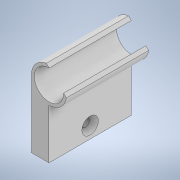
# Autodesk Inventor part: shadeHolderKetchenWindowV2
Saved by Autodesk Inventor 2022 (Build 260153070, 153G)
## iProperties
Created: 2021-02-12
Part Number: shadeHolderKetchenWindowV2
Material: Generic
Document SubType Name: Modeling
Designer: robst
Density: 1 g/cm^3
Appearance: Default
Author: robst
Autodesk Inventor part; units mm, degrees
ref_plane "YZ Plane" through (0, 0, 0) normal (1, 0, 0) x (0, 1, 0)
ref_plane "XZ Plane" through (0, 0, 0) normal (0, 1, 0) x (-1, 0, 0)
ref_plane "XY Plane" through (0, 0, 0) normal (0, 0, 1) x (1, 0, 0)
sketch "Sketch4" plane through (0, 0, 0) normal (0, 0, 1) x (1, 0, 0)
  arc A0 (0.0635, 6.3497) -> (6.3497, 0.0635) centre (0, 0) ccw
  arc A1 (-1.1235, 7.5367) -> (7.5367, -1.1235) centre (0, 0) ccw
  line L0 (0, 0) -> (0, 7.9375) construction
  line L1 (0.0635, 6.3497) -> (6.3497, 0.0635) construction
  line L2 (0.0635, 6.3497) -> (-1.1235, 7.5367)
  line L3 (6.3497, 0.0635) -> (7.5367, -1.1235)
  circle A2 centre (0, 0) radius 6.35
  dimension "d10" = 12.7
  dimension "d11" = 1.27
  dimension "d12" = 45
  dimension "d13" = 8.89
  constraints: 8 end point, 4 point on circle, 3 centre point, 3 coincident, 1 collinear, 1 concentric, 1 point on line, 1 vertical
  measures "d10" diameter of A0
  measures "d11" radial gap between concentric circles of A1 A0
  measures "d12" angle of L1 L0
  measures "d13" distance of L1.start L1.end
extrude "Extrusion3" add sketch "Sketch4" along normal mid plane 35.56 contours A0 L3 A1 L2
sketch "Sketch5" plane through (0, 0, 0) normal (0, 0, 1) x (1, 0, 0)
  arc A0 (-1.1235, 7.5367) -> (7.5367, -1.1235) centre (0, 0) ccw projected
  line L0 (-7.62, 0) -> (-7.62, -29.21)
  line L1 (-7.62, -29.21) -> (0, -29.21)
  line L2 (0, -29.21) -> (0, -7.62)
  circle A1 centre (0, 0) radius 7.9375
  dimension "d16" = 21.59
  constraints: 6 end point, 2 perpendicular, 2 point on circle, 1 centre point, 1 coincident, 1 tangent, 1 vertical
  measures "d16" distance from line of L2.end L1
extrude "Extrusion4" add sketch "Sketch5" along normal mid plane 35.56 contours A0 L2 A1 L0 | A1 L2 L1 L0 picked at (-7.3048, -2.4081)
sketch "Sketch6" plane through (0, -29.21, 17.78) normal (1, 0, 0) x (0, 0, -1)
  line L0 (0, 21.59) -> (35.56, 21.59) projected
  line L1 (35.56, 21.59) -> (35.56, 0) projected
  line L2 (0, 0) -> (35.56, 0) projected
  line L3 (0, 0) -> (0, 21.59) projected
  line L4 (17.78, 0) -> (17.78, 21.59) construction
  point P0 (17.78, 29.21)
  point P1 (17.78, 5.08)
  dimension "d30" = 5.08
  dimension "d31" = 0
  constraints: 2 end point, 2 midpoint
  measures "d30" distance from line of point (17.78, 5.08) L2
  measures "d31" distance from line of point (17.78, 5.08) L4
hole "Hole1" at (0, -24.13, 0) direction (-1, 0, 0) diameter 3.5052 end through all countersink diameter 7.112 countersink angle 82
sketch "Sketch10" plane through (-7.62, -29.21, 17.78) normal (0, -1, 0) x (1, 0, 0)
  line L0 (0, -35.56) -> (0, 0) projected
  line L1 (7.62, -35.56) -> (0, -35.56) projected
  line L2 (7.62, 0) -> (7.62, -35.56) projected
  line L3 (0, 0) -> (7.62, 0) projected
  line L4 (3.81, -35.56) -> (3.81, 0) construction
  line L5 (6.35, -29.5599) -> (1.27, -29.5599)
  line L6 (1.27, -29.5599) -> (1.27, -26.3818)
  line L7 (1.27, -26.3818) -> (1.871, -26.3818)
  line L8 (1.871, -26.3818) -> (1.871, -28.8848)
  line L9 (1.871, -28.8848) -> (3.2625, -28.8848)
  line L10 (3.2625, -28.8848) -> (3.2625, -26.5506)
  line L11 (3.2625, -26.5506) -> (3.8635, -26.5506)
  line L12 (3.8635, -26.5506) -> (3.8635, -28.8848)
  line L13 (3.8635, -28.8848) -> (5.749, -28.8848)
  line L14 (5.749, -28.8848) -> (5.749, -26.3818)
  line L15 (5.749, -26.3818) -> (6.35, -26.3818)
  line L16 (6.35, -26.3818) -> (6.35, -29.5599)
  line L17 (1.27, -19.9474) -> (6.35, -21.2236)
  line L18 (6.35, -21.2236) -> (6.35, -21.9811)
  line L19 (6.35, -21.9811) -> (2.1345, -23.0144)
  line L20 (2.1345, -23.0144) -> (6.35, -24.0188)
  line L21 (6.35, -24.0188) -> (6.35, -24.7681)
  line L22 (6.35, -24.7681) -> (1.27, -26.0648)
  line L23 (1.27, -26.0648) -> (1.27, -25.3691)
  line L24 (1.27, -25.3691) -> (5.4814, -24.3482)
  line L25 (5.4814, -24.3482) -> (1.27, -23.3355)
  line L26 (1.27, -23.3355) -> (1.27, -22.648)
  line L27 (1.27, -22.648) -> (5.5308, -21.6271)
  line L28 (5.5308, -21.6271) -> (1.27, -20.6102)
  line L29 (1.27, -20.6102) -> (1.27, -19.9474)
  line L30 (4.4357, -17.6256) -> (4.4357, -19.5481)
  line L31 (4.4357, -19.5481) -> (3.8182, -19.5481)
  line L32 (3.8182, -19.5481) -> (3.8182, -17.6256)
  line L33 (3.8182, -17.6256) -> (4.4357, -17.6256)
  spline S0 degree 2 poles (2.8014, -13.5954) (3.1307, -13.5954) (3.7235, -13.83) (3.9294, -14.04) knots 0 0 0 1 2 2 2
  spline S1 degree 2 poles (3.9294, -14.04) (4.1887, -14.3035) (4.4563, -15.0156) (4.4563, -15.559) knots 0 0 0 1 2 2 2
  line L34 (4.4563, -15.559) -> (4.4563, -16.1313)
  line L35 (4.4563, -16.1313) -> (6.35, -16.1313)
  line L36 (6.35, -16.1313) -> (6.35, -16.8064)
  line L37 (6.35, -16.8064) -> (1.27, -16.8064)
  line L38 (1.27, -16.8064) -> (1.27, -15.5302)
  spline S2 degree 2 poles (1.27, -15.5302) (1.27, -15.0774) (1.4182, -14.4434) (1.587, -14.2005) knots 0 0 0 1 2 2 2
  spline S3 degree 2 poles (1.587, -14.2005) (1.7805, -13.9165) (2.3774, -13.5954) (2.8014, -13.5954) knots 0 0 0 1 2 2 2
  spline S4 degree 2 poles (2.822, -14.2993) (2.5585, -14.2993) (2.1716, -14.4805) (2.0481, -14.6657) knots 0 0 0 1 2 2 2
  spline S5 degree 2 poles (2.0481, -14.6657) (1.941, -14.8263) (1.8546, -15.2544) (1.8546, -15.5714) knots 0 0 0 1 2 2 2
  line L39 (1.8546, -15.5714) -> (1.8546, -16.1313)
  line L40 (1.8546, -16.1313) -> (3.88, -16.1313)
  line L41 (3.88, -16.1313) -> (3.88, -15.6702)
  spline S6 degree 2 poles (3.88, -15.6702) (3.88, -15.2585) (3.7482, -14.7522) (3.5753, -14.5875) knots 0 0 0 1 2 2 2
  spline S7 degree 2 poles (3.5753, -14.5875) (3.423, -14.4352) (3.0649, -14.2993) (2.822, -14.2993) knots 0 0 0 1 2 2 2
  line L42 (1.27, -9.2687) -> (6.35, -11.0183)
  line L43 (6.35, -11.0183) -> (6.35, -11.747)
  line L44 (6.35, -11.747) -> (1.27, -13.4966)
  line L45 (1.27, -13.4966) -> (1.27, -12.772)
  line L46 (1.27, -12.772) -> (5.4896, -11.3641)
  line L47 (5.4896, -11.3641) -> (1.27, -9.9562)
  line L48 (1.27, -9.9562) -> (1.27, -9.2687)
  line L49 (6.35, -5.9918) -> (6.35, -8.4701)
  line L50 (6.35, -8.4701) -> (5.8313, -8.4701)
  line L51 (5.8313, -8.4701) -> (5.8313, -7.548)
  line L52 (5.8313, -7.548) -> (2.4268, -7.548)
  line L53 (2.4268, -7.548) -> (2.4268, -8.4701)
  line L54 (2.4268, -8.4701) -> (1.9616, -8.4701)
  spline S8 degree 2 poles (1.9616, -8.4701) (1.9616, -7.9473) (1.6652, -7.4533) (1.2535, -7.4203) knots 0 0 0 1 2 2 2
  line L55 (1.2535, -7.4203) -> (1.2535, -6.8934)
  line L56 (1.2535, -6.8934) -> (5.8313, -6.8934)
  line L57 (5.8313, -6.8934) -> (5.8313, -5.9918)
  line L58 (5.8313, -5.9918) -> (6.35, -5.9918)
  point P0 (7.62, -17.78)
  constraints: 2 end point, 2 midpoint, 1 vertical
extrude "Text" cut sketch "Sketch10" against normal blind 1.143 contours L5 L6 L7 L8 L9 L10 L11 L12 L13 L14 L15 L16 | L17 L18 L19 L20 L21 L22 L23 L24 L25 L26 L27 L28 L29 | L30 L31 L32 L33 | S0 S1 L34 L35 L36 L37 L38 S2 S3 | L42 L43 L44 L45 L46 L47 L48 | L49 L50 L51 L52 L53 L54 S8 L55 L56 L57 L58
equation "\"d10\" = shadeDiameter"
equation "\"d11\" = shadeHolderWallThickness"
equation "\"d13\" = openingForShade"
equation "\"d14\" = partWidth"
equation "\"d16\" = flatBelowShade"
equation "\"d17\" = partWidth"
equation "\"d30\" = holeHeightAboveBottom"
equation "\"d28\" = textDepth"
equation "\"shadeDiameter\" = 12.7"
equation "\"partWidth\" = 35.56"
equation "\"backThickness\" = 1.905"
equation "\"backHeight\" = 25.4"
equation "\"cutTiltAngle\" = 45deg"
equation "\"flatBelowShade\" = 21.59"
equation "\"shadeHolderWallThickness\" = 1.27"
equation "\"openingForShade\" = 8.89"
equation "\"textDepth\" = 1.143"
equation "\"holeHeightAboveBottom\" = 5.08"
body "Solid2"
